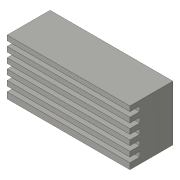
# Autodesk Inventor part: Victor2
Saved by Autodesk Inventor 2016 (Build 200138000, 138)
## iProperties
Created: 2016-01-27
Part Number: Victor2
Material: Generic
Document SubType Name: Modeling
Designer: PrashantBIA
Density: 1 g/cm^3
Appearance: Light Gray
Author: PrashantBIA
Autodesk Inventor part; units mm, degrees
ref_plane "YZ Plane" through (0, 0, 0) normal (1, 0, 0) x (0, 1, 0)
ref_plane "XZ Plane" through (0, 0, 0) normal (0, 1, 0) x (-1, 0, 0)
ref_plane "XY Plane" through (0, 0, 0) normal (0, 0, 1) x (1, 0, 0)
sketch "Sketch1" plane through (0, 0, 0) normal (0, 0, 1) x (1, 0, 0)
  line L0 (0, 0) -> (63.5, 0)
  line L1 (63.5, 0) -> (63.5, 28.575)
  line L2 (63.5, 28.575) -> (0, 28.575)
  line L3 (0, 28.575) -> (0, 0)
  dimension "d0" = 63.5
  dimension "d1" = 28.575
  constraints: 8 end point, 2 parallel, 1 horizontal, 1 perpendicular
  measures "d0" distance of L1.end L2.end
  measures "d1" distance of L2.end L0.start
extrude "Extrusion1" add sketch "Sketch1" along normal blind 22.225
sketch "Sketch2" plane through (0, 0, 22.225) normal (0, 0, 1) x (1, 0, 0)
  line L0 (63.5, 0) -> (63.5, 28.575) projected
  line L1 (0, 28.575) -> (0, 0) projected
  line L2 (63.5, 26.035) -> (0, 26.035)
  line L3 (0, 26.035) -> (0, 23.495)
  line L4 (0, 23.495) -> (63.5, 23.495)
  line L5 (63.5, 23.495) -> (63.5, 26.035)
  line L6 (63.5, 28.575) -> (0, 28.575) projected
  line L7 (63.5, 20.955) -> (0, 20.955)
  line L8 (0, 20.955) -> (0, 18.415)
  line L9 (0, 18.415) -> (63.5, 18.415)
  line L10 (63.5, 18.415) -> (63.5, 20.955)
  line L11 (63.5, 15.875) -> (0, 15.875)
  line L12 (0, 15.875) -> (0, 13.335)
  line L13 (0, 13.335) -> (63.5, 13.335)
  line L14 (63.5, 13.335) -> (63.5, 15.875)
  line L15 (63.5, 10.795) -> (0, 10.795)
  line L16 (0, 10.795) -> (0, 8.255)
  line L17 (0, 8.255) -> (63.5, 8.255)
  line L18 (63.5, 8.255) -> (63.5, 10.795)
  line L19 (63.5, 5.715) -> (0, 5.715)
  line L20 (0, 5.715) -> (0, 3.175)
  line L21 (0, 3.175) -> (63.5, 3.175)
  line L22 (63.5, 3.175) -> (63.5, 5.715)
  dimension "d4" = 2.54
  dimension "d5" = 2.54
  dimension "d8" = 5.08
  constraints: 40 end point, 2 parallel, 2 point on line, 1 horizontal, 1 perpendicular, 1 vertical, 32 other
  measures "d4" distance between parallel lines of L4 L2
  measures "d5" distance between parallel lines of L2 L6
  measures "d8" distance of L2.start L7.start
extrude "Extrusion2" cut sketch "Sketch2" against normal blind 5.08 contours L21 L1 L19 L0 | L17 L1 L15 L0 | L13 L1 L11 L0 | L9 L1 L7 L0 | L4 L1 L2 L0
body "Solid1"
